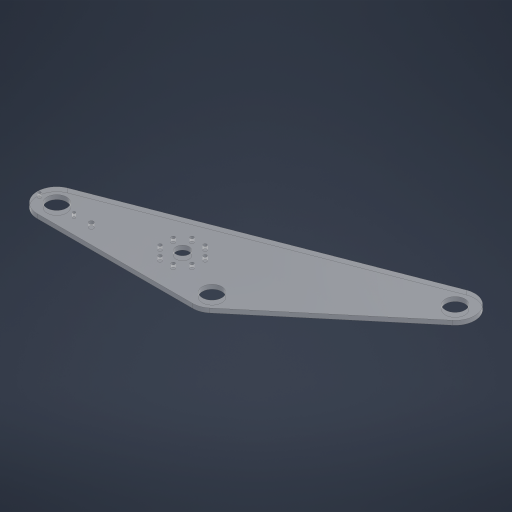
# Autodesk Inventor part: CORL_006_SmallPlate
Saved by Autodesk Inventor 2024.2 (Build 282272000, 272)
## iProperties
Created: 2024-08-02
Part Number: CORL_006_SmallPlate
Material: Polycarbonate, Clear
Document SubType Name: Modeling
Designer: Bryan
Density: 1.2 g/cm^3
Appearance: Polycarbonate - Clear
Mass: 347.539 g
Surface Area: 1011.9 cm^2
Volume: 289.616 cm^3
Author: Bryan
Autodesk Inventor part; units mm, degrees
ref_plane "YZ Plane" through (0, 0, 0) normal (1, 0, 0) x (0, 1, 0)
ref_plane "XZ Plane" through (0, 0, 0) normal (0, 1, 0) x (-1, 0, 0)
ref_plane "XY Plane" through (0, 0, 0) normal (0, 0, 1) x (1, 0, 0)
sketch "Sketch1" plane through (0, 0, 0) normal (0, 1, 0) x (-1, 0, 0)
  circle A0 centre (0, 0) radius 14.2875
  line L0 (0, 0) -> (228.6, 0) construction
  circle A1 centre (228.6, 0) radius 14.2875
  circle A2 centre (0, 0) radius 28.575 construction
  circle A3 centre (228.6, 0) radius 28.575 construction
  line L1 (228.6, -28.575) -> (0, -28.575)
  line L2 (0, 28.575) -> (228.6, 28.575)
  arc A4 (228.6, -28.575) -> (228.6, 28.575) centre (228.6, 0) ccw
  arc A5 (0, 28.575) -> (0, -28.575) centre (0, 0) ccw
  dimension "d0" = 28.575
  dimension "d1" = 228.6
  dimension "d5" = 57.15
  constraints: 8 point on circle, 7 tangent, 6 centre point, 6 end point, 4 coincident, 2 equal radius, 1 horizontal
  measures "d0" diameter of A0
  measures "d1" distance of L0.start L0.end
  measures "d5" diameter of A2
extrude "Extrusion1" add sketch "Sketch1" along normal blind 6.35
sketch "Sketch3" plane through (0, 6.35, 0) normal (0, 1, 0) x (1, 0, 0)
  circle A0 centre (-228.6, 0) radius 14.2875 construction
  line L0 (0, 0) -> (-228.6, 0) construction
  circle A1 centre (0, 0) radius 14.2875 construction
  line L1 (0, 0) -> (194.5753, 163.2681) construction
  arc A2 (0, -28.575) -> (0, 28.575) centre (0, 0) ccw projected
  circle A3 centre (0, 0) radius 28.575
  circle A4 centre (194.5753, 163.2681) radius 28.575 construction
  circle A5 centre (194.5753, 163.2681) radius 14.2875
  circle A6 centre (0, 0) radius 14.2875 projected
  line L2 (176.2076, 185.1578) -> (-18.3677, 21.8897)
  line L3 (212.9429, 141.3783) -> (18.3677, -21.8897)
  arc A7 (212.9429, 141.3783) -> (176.2076, 185.1578) centre (194.5753, 163.2681) ccw
  point P0 (0, 28.575)
  point P1 (18.3677, -21.8897)
  dimension "d12" = 254
  dimension "d13" = 140
  constraints: 8 end point, 7 point on circle, 5 tangent, 4 centre point, 3 coincident, 2 equal radius, 1 horizontal
  measures "d12" distance of L1.start L1.end
  measures "d13" angle of L0 L1
extrude "Extrusion3" add sketch "Sketch3" against normal blind 6.35 contours A2 A3 L2 A7 L3
sketch "Sketch4" plane through (0, 6.35, 0) normal (0, 1, 0) x (1, 0, 0)
  circle A0 centre (-74.9321, 31.4901) radius 30 construction
  circle A1 centre (-74.9321, 31.4901) radius 25.4 construction
  circle A2 centre (-74.9321, 31.4901) radius 9.6012
  circle A3 centre (0, 0) radius 40.64 construction
  circle A4 centre (-74.9321, 31.4901) radius 40.64 construction
  line L0 (-84.6522, 8.0235) -> (-84.6522, 54.9566) construction
  line L1 (-84.6522, 54.9566) -> (-65.2119, 54.9566) construction
  line L2 (-65.2119, 54.9566) -> (-65.2119, 8.0235) construction
  line L3 (-65.2119, 8.0235) -> (-84.6522, 8.0235) construction
  circle A5 centre (-84.6522, 8.0235) radius 2.4892
  circle A6 centre (-65.2119, 8.0235) radius 2.4892
  circle A7 centre (-51.4655, 21.7699) radius 2.4892
  circle A8 centre (-51.4655, 41.2102) radius 2.4892
  line L4 (2.5406, 40.5605) -> (-2.5406, -40.5605) construction
  circle A9 centre (194.5753, 163.2681) radius 14.2875 construction
  line L5 (-74.9321, 31.4901) -> (194.5753, 163.2681) construction
  circle A10 centre (194.5753, 163.2681) radius 14.2875 projected
  circle A11 centre (0, 0) radius 14.2875 projected
  circle A12 centre (-228.6, 0) radius 14.2875 projected
  line L6 (-10.4004, 28.575) -> (-228.6, 28.575) projected
  arc A13 (-228.6, 28.575) -> (-228.6, -28.575) centre (-228.6, 0) ccw projected
  line L7 (-228.6, -28.575) -> (0, -28.575) projected
  arc A14 (0, -28.575) -> (18.3677, -21.8897) centre (0, 0) ccw projected
  line L8 (18.3677, -21.8897) -> (212.9429, 141.3783) projected
  arc A15 (212.9429, 141.3783) -> (176.2076, 185.1578) centre (194.5753, 163.2681) ccw projected
  line L9 (176.2076, 185.1578) -> (-10.4004, 28.575) projected
  arc A16 (-228.6, 28.575) -> (-228.6, -28.575) centre (-228.6, 0) ccw projected
  circle A17 centre (0, 0) radius 50.8 construction
  arc A18 (-228.6, 28.575) -> (-228.6, -28.575) centre (-228.6, 0) ccw projected
  arc A19 (212.9429, 141.3783) -> (176.2076, 185.1578) centre (194.5753, 163.2681) ccw projected
  line L10 (-238.8857, 26.6596) -> (184.2896, 189.9277)
  circle A20 centre (-65.2119, 54.9566) radius 2.4892
  circle A21 centre (-84.6522, 54.9566) radius 2.4892
  circle A22 centre (-98.3986, 41.2102) radius 2.4892
  circle A23 centre (-98.3986, 21.7699) radius 2.4892
  point P0 (34.7284, 53.046)
  point P1 (38.9386, 55.4768)
  point P2 (-93.3302, 28.575)
  point P3 (-88.3521, 28.575)
  point P4 (-73.8899, 28.575)
  point P5 (-68.9118, 28.575)
  point P6 (-75.3508, 28.575)
  point P7 (-71.7292, 28.575)
  point P8 (-55.9105, 28.575)
  point P9 (-52.2889, 28.575)
  dimension "d16" = 60
  dimension "d17" = 50.8
  dimension "d18" = 19.2024
  dimension "d19" = 81.28
  dimension "d21" = 4.9784
  dimension "d24" = 360
  dimension "d26" = 299.9994
  dimension "d31" = 101.6
  constraints: 14 centre point, 14 end point, 9 coincident, 7 point on circle, 3 parallel, 3 tangent, 1 equal radius, 1 perpendicular, 23 other
  measures "d16" diameter of A0
  measures "d17" diameter of A1
  measures "d18" diameter of A2
  measures "d19" diameter of A3
  measures "d21" diameter of A5
  measures "d26" distance of L5.start L5.end
  measures "d31" diameter of A17
extrude "Extrusion7" cut sketch "Sketch4" against normal blind 6.35 contours A2 L6 | L6 A2 | A5 | A6 | A7 | A8 | A20 | A21 | A22 | A23
extrude "Extrusion8" add sketch "Sketch4" against normal blind 6.35 contours A2 L6 A13 L10 A15 L9
sketch "Sketch5" plane through (0, 6.35, 0) normal (0, 1, 0) x (1, 0, 0)
  line L0 (-238.8857, 26.6596) -> (184.2896, 189.9277) projected
  circle A0 centre (68.7646, 145.3562) radius 15.875
  point P0 (0, 0)
  dimension "d38" = 31.75
  dimension "d41" = 123.825
  constraints: 1 centre point, 1 point on line
  measures "d38" diameter of A0
  measures "d41" distance of A0.centre L0.end
extrude "Extrusion9" [suppressed]
fillet "Fillet1" [suppressed]
sketch "Sketch6" plane through (0, 6.35, 0) normal (0, 1, 0) x (1, 0, 0)
  circle A0 centre (-228.6, 0) radius 14.2875 construction
  line L0 (-228.6, 0) -> (-177.8, 0) construction
  circle A1 centre (-177.8, 0) radius 3.2512
  point P0 (0, 0)
  dimension "d43" = 50.8
  dimension "d44" = 6.5024
  constraints: 2 end point, 1 centre point, 1 coincident, 1 horizontal
  measures "d43" distance of L0.start L0.end
  measures "d44" diameter of A1
extrude "Extrusion10" cut sketch "Sketch6" against normal blind 6.35
sketch "Sketch7" plane through (0, 6.35, 0) normal (0, 1, 0) x (1, 0, 0)
  circle A0 centre (-254, 0) radius 1.9812
  circle A1 centre (-203.2, 0) radius 1.9812
  line L0 (-203.2, 0) -> (-254, 0) construction
  circle A2 centre (-228.6, 0) radius 14.2875 construction
  point P0 (0, 0)
  dimension "d47" = 50.8
  dimension "d48" = 3.9624
  constraints: 2 centre point, 2 end point, 1 coincident, 1 equal radius, 1 horizontal, 1 midpoint
  measures "d47" distance of L0.start L0.end
  measures "d48" diameter of A1
extrude "Extrusion11" cut sketch "Sketch7" against normal blind 6.35
body "Solid1"
